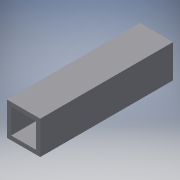
# Autodesk Inventor part: flywheelsupport
Saved by Autodesk Inventor 2016 (Build 200138000, 138)
## iProperties
Created: 2016-01-29
Part Number: flywheelsupport
Material: Generic
Document SubType Name: Modeling
Designer: zachary
Density: 1 g/cm^3
Appearance: Default
Mass: 45.0644 g
Surface Area: 292.741 cm^2
Volume: 45.0644 cm^3
Author: zachary
Autodesk Inventor part; units mm, degrees
ref_plane "YZ Plane" through (0, 0, 0) normal (1, 0, 0) x (0, 1, 0)
ref_plane "XZ Plane" through (0, 0, 0) normal (0, 1, 0) x (-1, 0, 0)
ref_plane "XY Plane" through (0, 0, 0) normal (0, 0, 1) x (1, 0, 0)
sketch "Sketch1" plane through (0, 0, 0) normal (0, 0, 1) x (1, 0, 0)
  line L0 (0, 0) -> (25.4, 0)
  line L1 (25.4, 0) -> (25.4, -25.4)
  line L2 (25.4, -25.4) -> (0, -25.4)
  line L3 (0, -25.4) -> (0, 0)
  line L4 (3.175, -3.175) -> (22.225, -3.175)
  line L5 (22.225, -3.175) -> (22.225, -22.225)
  line L6 (22.225, -22.225) -> (3.175, -22.225)
  line L7 (3.175, -22.225) -> (3.175, -3.175)
  dimension "d0" = 25.4
  dimension "d1" = 25.4
  dimension "d2" = 3.175
  dimension "d3" = 3.175
  dimension "d4" = 3.175
  dimension "d5" = 3.175
  constraints: 16 end point, 4 parallel, 2 horizontal, 2 perpendicular
  measures "d0" distance between parallel lines of L3 L1
  measures "d1" distance between parallel lines of L0 L2
  measures "d2" distance between parallel lines of L1 L5
  measures "d3" distance between parallel lines of L2 L6
  measures "d4" distance between parallel lines of L3 L7
  measures "d5" distance between parallel lines of L0 L4
extrude "Extrusion1" add sketch "Sketch1" along normal blind 101.6
sketch "Sketch2" plane through (25.4, -25.4, 0) normal (1, 0, 0) x (0, 0, -1)
  circle A0 centre (-63.5, 12.7) radius 3.3734
  line L0 (0, 25.4) -> (0, 0) projected
  line L1 (0, 25.4) -> (-101.6, 25.4) projected
  circle A1 centre (-88.9, 12.7) radius 3.3734
  dimension "d8" = 6.7469
  dimension "d12" = 63.5
  dimension "d13" = 88.9
  dimension "d14" = 12.7
  dimension "d17" = 12.7
  constraints: 2 centre point, 1 equal radius
  measures "d8" diameter of A0
  measures "d12" distance from line of L0 A0.centre
  measures "d13" distance from line of L0 A1.centre
  measures "d14" distance from line of L1 A1.centre
  measures "d17" distance from line of L1 A0.centre
extrude "Extrusion3" cut sketch "Sketch2" against normal blind 25.4
body "Solid1"
